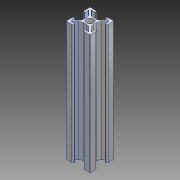
# Autodesk Inventor part: Perfil 20 x 20 Básico - LEGP20101
Saved by Autodesk Inventor 2016 (Build 200138000, 138)
## iProperties
Created: 2016-04-02
Part Number: Perfil 20 x 20 Básico - LEGP20101
Material: Aluminum 6061
Document SubType Name: Modeling
Designer: Vinicius
Density: 2.7 g/cm^3
Appearance: Aluminum - Flat
Author: Vinicius
Autodesk Inventor part; units mm, degrees
ref_plane "YZ Plane" through (0, 0, 0) normal (1, 0, 0) x (0, 1, 0)
ref_plane "XZ Plane" through (0, 0, 0) normal (0, 1, 0) x (-1, 0, 0)
ref_plane "XY Plane" through (0, 0, 0) normal (0, 0, 1) x (1, 0, 0)
sketch "Sketch1" plane through (0, 0, 0) normal (0, 0, 1) x (1, 0, 0)
  line L0 (-4.1988, 5.1716) -> (-7.1858, 8.1586)
  arc A0 (-7.0444, 8.5) -> (-7.1858, 8.1586) centre (-7.0444, 8.3) ccw
  line L1 (-7.0444, 8.5) -> (-4.15, 8.5)
  line L2 (-4.15, 8.5) -> (-4.15, 9)
  arc A1 (-4.15, 9) -> (-5.15, 10) centre (-5.15, 9) ccw
  line L3 (-5.15, 10) -> (-9.6, 10)
  arc A2 (-9.6, 10) -> (-10, 9.6) centre (-9.6, 9.6) ccw
  line L4 (-10, 9.6) -> (-10, 5.15)
  arc A3 (-10, 5.15) -> (-9, 4.15) centre (-9, 5.15) ccw
  line L5 (-9, 4.15) -> (-8.5, 4.15)
  line L6 (-8.5, 4.15) -> (-8.5, 7.0444)
  arc A4 (-8.1586, 7.1858) -> (-8.5, 7.0444) centre (-8.3, 7.0444) ccw
  line L7 (-8.1586, 7.1858) -> (-5.1716, 4.1988)
  arc A5 (-4, 1.3704) -> (-5.1716, 4.1988) centre (-8, 1.3704) ccw
  line L8 (-4, 1.3704) -> (-4, 0)
  line L9 (-4, 0) -> (-4, -1.3704)
  arc A6 (-5.1716, -4.1988) -> (-4, -1.3704) centre (-8, -1.3704) ccw
  line L10 (-5.1716, -4.1988) -> (-8.1586, -7.1858)
  arc A7 (-8.5, -7.0444) -> (-8.1586, -7.1858) centre (-8.3, -7.0444) ccw
  line L11 (-8.5, -7.0444) -> (-8.5, -4.15)
  line L12 (-8.5, -4.15) -> (-9, -4.15)
  arc A8 (-9, -4.15) -> (-10, -5.15) centre (-9, -5.15) ccw
  line L13 (-10, -5.15) -> (-10, -9.6)
  arc A9 (-10, -9.6) -> (-9.6, -10) centre (-9.6, -9.6) ccw
  line L14 (-9.6, -10) -> (-5.15, -10)
  arc A10 (-5.15, -10) -> (-4.15, -9) centre (-5.15, -9) ccw
  line L15 (-4.15, -9) -> (-4.15, -8.5)
  line L16 (-4.15, -8.5) -> (-7.0444, -8.5)
  arc A11 (-7.1858, -8.1586) -> (-7.0444, -8.5) centre (-7.0444, -8.3) ccw
  line L17 (-7.1858, -8.1586) -> (-4.1988, -5.1716)
  arc A12 (-1.3704, -4) -> (-4.1988, -5.1716) centre (-1.3704, -8) ccw
  line L18 (-1.3704, -4) -> (0, -4)
  line L19 (0, -4) -> (1.3704, -4)
  arc A13 (4.1988, -5.1716) -> (1.3704, -4) centre (1.3704, -8) ccw
  line L20 (4.1988, -5.1716) -> (7.1858, -8.1586)
  arc A14 (7.0444, -8.5) -> (7.1858, -8.1586) centre (7.0444, -8.3) ccw
  line L21 (7.0444, -8.5) -> (4.15, -8.5)
  line L22 (4.15, -8.5) -> (4.15, -9)
  arc A15 (4.15, -9) -> (5.15, -10) centre (5.15, -9) ccw
  line L23 (5.15, -10) -> (9.6, -10)
  arc A16 (9.6, -10) -> (10, -9.6) centre (9.6, -9.6) ccw
  line L24 (10, -9.6) -> (10, -5.15)
  arc A17 (10, -5.15) -> (9, -4.15) centre (9, -5.15) ccw
  line L25 (9, -4.15) -> (8.5, -4.15)
  line L26 (8.5, -4.15) -> (8.5, -7.0444)
  arc A18 (8.1586, -7.1858) -> (8.5, -7.0444) centre (8.3, -7.0444) ccw
  line L27 (8.1586, -7.1858) -> (5.1716, -4.1988)
  arc A19 (4, -1.3704) -> (5.1716, -4.1988) centre (8, -1.3704) ccw
  line L28 (4, -1.3704) -> (4, 0)
  line L29 (4, 0) -> (4, 1.3704)
  arc A20 (5.1716, 4.1988) -> (4, 1.3704) centre (8, 1.3704) ccw
  line L30 (5.1716, 4.1988) -> (8.1586, 7.1858)
  arc A21 (8.5, 7.0444) -> (8.1586, 7.1858) centre (8.3, 7.0444) ccw
  line L31 (8.5, 7.0444) -> (8.5, 4.15)
  line L32 (8.5, 4.15) -> (9, 4.15)
  arc A22 (9, 4.15) -> (10, 5.15) centre (9, 5.15) ccw
  line L33 (10, 5.15) -> (10, 9.6)
  arc A23 (10, 9.6) -> (9.6, 10) centre (9.6, 9.6) ccw
  line L34 (9.6, 10) -> (5.15, 10)
  arc A24 (5.15, 10) -> (4.15, 9) centre (5.15, 9) ccw
  line L35 (4.15, 9) -> (4.15, 8.5)
  line L36 (4.15, 8.5) -> (7.0444, 8.5)
  arc A25 (7.1858, 8.1586) -> (7.0444, 8.5) centre (7.0444, 8.3) ccw
  line L37 (7.1858, 8.1586) -> (4.1988, 5.1716)
  arc A26 (1.3704, 4) -> (4.1988, 5.1716) centre (1.3704, 8) ccw
  line L38 (1.3704, 4) -> (0, 4)
  line L39 (0, 4) -> (-1.3704, 4)
  arc A27 (-4.1988, 5.1716) -> (-1.3704, 4) centre (-1.3704, 8) ccw
  circle A28 centre (0, 0) radius 3.05
  constraints: 80 end point, 56 point on circle, 29 centre point
extrude "Extrusion1" add sketch "Sketch1" along normal mid plane 100
body "Solid1"
